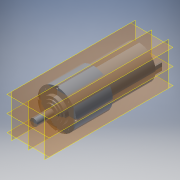
# Autodesk Inventor part: Drive Motor
Saved by Autodesk Inventor 2016 (Build 200138000, 138)
## iProperties
Created: 2016-03-03
Part Number: Drive Motor
Material: Generic
Document SubType Name: Modeling
Designer: Spencer
Density: 1 g/cm^3
Appearance: Default
Mass: 48.7353 g
Surface Area: 88.2482 cm^2
Volume: 48.7353 cm^3
Author: Spencer
Autodesk Inventor part; units mm, degrees
ref_plane "XZ Plane" through (0, 0, 0) normal (0, 1, 0) x (-1, 0, 0)
sketch "Sketch1" plane through (0, 0, 0) normal (0, 1, 0) x (-1, 0, 0)
  circle A0 centre (0, 0) radius 16
  dimension "d0" = 32
  constraints: 1 centre point, 1 coincident
  measures "d0" diameter of A0
extrude "Extrusion1" add sketch "Sketch1" along normal blind 30.4
sketch "Sketch2" plane through (0, 30.4, 0) normal (0, 1, 0) x (1, 0, 0)
  circle A0 centre (0, 0) radius 13.75
  dimension "d3" = 27.5
  constraints: 1 centre point, 1 coincident
  measures "d3" diameter of A0
extrude "Extrusion2" add sketch "Sketch2" along normal blind 37.8
sketch "Sketch3" plane through (0, 0, 0) normal (0, -1, 0) x (1, 0, 0)
  circle A0 centre (0, 0) radius 10
  dimension "d6" = 20
  constraints: 1 centre point, 1 coincident
  measures "d6" diameter of A0
extrude "Extrusion3" add sketch "Sketch3" along normal blind 3
sketch "Sketch4" plane through (0, -3, 0) normal (0, -1, 0) x (1, 0, 0)
  circle A0 centre (0, 0) radius 8
  dimension "d9" = 16
  constraints: 1 centre point, 1 coincident
  measures "d9" diameter of A0
extrude "Extrusion4" add sketch "Sketch4" along normal blind 1
sketch "Sketch5" plane through (0, -4, 0) normal (0, -1, 0) x (1, 0, 0)
  circle A0 centre (0, 0) radius 6
  dimension "d12" = 12
  constraints: 1 centre point, 1 coincident
  measures "d12" diameter of A0
extrude "Extrusion5" add sketch "Sketch5" along normal blind 1
sketch "Sketch6" plane through (0, -5, 0) normal (0, -1, 0) x (1, 0, 0)
  circle A0 centre (0, 0) radius 3
  dimension "d15" = 6
  constraints: 1 centre point, 1 coincident
  measures "d15" diameter of A0
extrude "Extrusion6" add sketch "Sketch6" along normal blind 14.3
sketch "Sketch7" plane through (0, 68.2, 0) normal (0, 1, 0) x (1, 0, 0)
  line L0 (-9.25, -6) -> (-10.75, -6)
  line L1 (-10.75, -6) -> (-10.75, 6)
  line L2 (-10.75, 6) -> (-9.25, 6)
  line L3 (-9.25, 6) -> (-9.25, -6)
  circle A0 centre (0, 0) radius 10 projected
  line L4 (-9.25, -6) -> (-10.75, 6) construction
  line L5 (-10.75, -6) -> (-9.25, 6) construction
  point P0 (-10, 0)
  dimension "d18" = 12
  dimension "d19" = 1.5
  constraints: 12 end point, 2 midpoint, 2 parallel, 1 horizontal, 1 horizontal alignment, 1 perpendicular, 1 other
  measures "d18" distance of L0.end L1.end
  measures "d19" distance of L1.end L2.end
extrude "Extrusion7" [suppressed]
sketch "Sketch8" plane through (-10.75, 68.2, -6) normal (-1, 0, 0) x (0, 0, 1)
  line L0 (1.5, 11.5) -> (10.5, 11.5)
  line L1 (10.5, 11.5) -> (10.5, 8.812)
  line L2 (10.5, 8.812) -> (1.5, 8.812)
  line L3 (1.5, 8.812) -> (1.5, 11.5)
  line L4 (0, 12.5) -> (12, 12.5) projected
  line L5 (0, 0) -> (0, 12.5) projected
  line L6 (12, 0) -> (12, 12.5) projected
  point P0 (6, -68.2)
  dimension "d22" = 1
  dimension "d23" = 1.5
  dimension "d24" = 1.5
  constraints: 8 end point, 2 parallel, 1 horizontal, 1 perpendicular
  measures "d22" distance from line of L0.start L4
  measures "d23" distance from line of L0.start L5
  measures "d24" distance from line of L0.end L6
extrude "Extrusion8" [suppressed]
sketch "Sketch9" plane through (0, 0, 0) normal (0, -1, 0) x (1, 0, 0)
  circle A0 centre (0, 0) radius 13.75 projected
  line L0 (-9.4443, 9.9933) -> (9.4443, 9.9933)
  line L1 (9.4443, 9.9933) -> (9.4443, -9.9933)
  line L2 (9.4443, -9.9933) -> (-9.4443, -9.9933)
  line L3 (-9.4443, -9.9933) -> (-9.4443, 9.9933)
  line L4 (-9.4443, 9.9933) -> (9.4443, -9.9933) construction
  line L5 (9.4443, 9.9933) -> (-9.4443, -9.9933) construction
  circle A1 centre (9.4443, -9.9933) radius 0.5
  circle A2 centre (-9.4443, -9.9933) radius 0.5
  circle A3 centre (-9.4443, 9.9933) radius 0.5
  circle A4 centre (9.4443, 9.9933) radius 0.5
  dimension "d27" = 1
  dimension "d28" = 1
  dimension "d29" = 1
  dimension "d30" = 1
  constraints: 12 end point, 4 centre point, 4 coincident, 2 midpoint, 2 parallel, 1 horizontal, 1 perpendicular, 2 other
  measures "d27" diameter of A1
  measures "d28" diameter of A2
  measures "d29" diameter of A3
  measures "d30" diameter of A4
extrude "Extrusion9" cut sketch "Sketch9" against normal blind 1 contours A4 L1 A0 | A0 A4 | A1 A0 | A0 L1 A1 | L0 A4 A0 | L1 A4 L0 | L2 A1 L1 | A0 A1 L2 | A3 L0 A0 | A0 A3 | A3 L3 L0 | A2 A0 | A0 L2 A2 | L2 L3 A2 | L3 A3 A0 | A0 A2 L3
sketch "Sketch10" plane through (0, 0, 0) normal (0, -1, 0) x (1, 0, 0)
  circle A0 centre (0, 0) radius 16 projected
  line L0 (0, 16) -> (0, 14.5)
  line L1 (0, 14.5) -> (-1, 14.5)
  line L2 (-1, 14.5) -> (-1, 16)
  line L3 (-1, 16) -> (0, 16)
  line L4 (0, 16) -> (0, 14.5)
  line L5 (0, 14.5) -> (1, 14.5)
  line L6 (1, 14.5) -> (1, 16)
  line L7 (1, 16) -> (0, 16)
  dimension "d33" = 1
  dimension "d34" = 1
  dimension "d35" = 1.5
  constraints: 16 end point, 5 equal length, 2 perpendicular, 1 vertical, 1 vertical alignment, 1 other
  measures "d33" distance of L0.end L1.end
  measures "d34" distance of L0.end L5.end
  measures "d35" distance of L0.start L0.end
extrude "Extrusion10" cut sketch "Sketch10" against normal blind 1 contours L6 L5 L0 A0 | A0 L7 L6 | L2 L3 A0 | A0 L0 L1 L2
mirror "Mirror1" about plane through (0, 0, 0) normal (0, 0, 1) of "Extrusion10"
sketch "Sketch11" plane through (0, 0, 0) normal (0, -1, 0) x (1, 0, 0)
  arc A0 (1, -15.9687) -> (1, 15.9687) centre (0, 0) ccw projected
  line L0 (16, 0) -> (14.5, 0)
  line L1 (14.5, 0) -> (14.5, 1)
  line L2 (14.5, 1) -> (16, 1)
  line L3 (16, 1) -> (16, 0)
  line L4 (16, 0) -> (14.5, 0)
  line L5 (14.5, 0) -> (14.5, -1)
  line L6 (14.5, -1) -> (16, -1)
  line L7 (16, -1) -> (16, 0)
  dimension "d38" = 1
  dimension "d39" = 1
  dimension "d40" = 1.5
  constraints: 16 end point, 4 parallel, 3 perpendicular, 1 horizontal, 1 point on circle
  measures "d38" distance of L0.end L5.end
  measures "d39" distance of L0.end L1.end
  measures "d40" distance of L0.start L0.end
extrude "Extrusion11" cut sketch "Sketch11" against normal blind 1
mirror "Mirror2" about plane through (0, 0, 0) normal (1, 0, 0) of "Extrusion11"
sketch "Sketch12" plane through (0, 68.2, 0) normal (0, 1, 0) x (1, 0, 0)
  line L0 (-13.0359, 2.9472) -> (-13.0359, -2.9472)
  line L1 (-13.0359, -2.9472) -> (-11.9023, -2.9472)
  line L2 (-11.9023, -2.9472) -> (-11.9023, 2.9472)
  line L3 (-11.9023, 2.9472) -> (-13.0359, 2.9472)
  line L4 (-13.0359, 2.9472) -> (-11.9023, -2.9472) construction
  line L5 (-13.0359, -2.9472) -> (-11.9023, 2.9472) construction
  point P0 (0, 0)
  point P1 (-12.4691, 0)
  constraints: 12 end point, 2 midpoint, 2 parallel, 1 perpendicular, 1 vertical
extrude "Extrusion12" add sketch "Sketch12" along normal blind 6
ref_plane "Work Plane1" through (0, 30.4, 13.75) normal (0, 0, 1) x (1, 0, 0)
ref_plane "Work Plane3" through (0, 30.4, 0) normal (0, 0, 1) x (1, 0, 0)
ref_plane "Work Plane2" through (0, 30.4, -13.75) normal (0, 0, 1) x (1, 0, 0)
ref_plane "Work Plane4" through (-13.75, 30.4, 0) normal (1, 0, 0) x (0, 1, 0)
ref_plane "Work Plane6" through (0, 30.4, 0) normal (1, 0, 0) x (0, 1, 0)
ref_plane "Work Plane5" through (13.75, 30.4, 0) normal (1, 0, 0) x (0, 1, 0)
mirror "Mirror3" about plane through (0, 30.4, 0) normal (1, 0, 0) of "Extrusion12"
body "Solid1"
